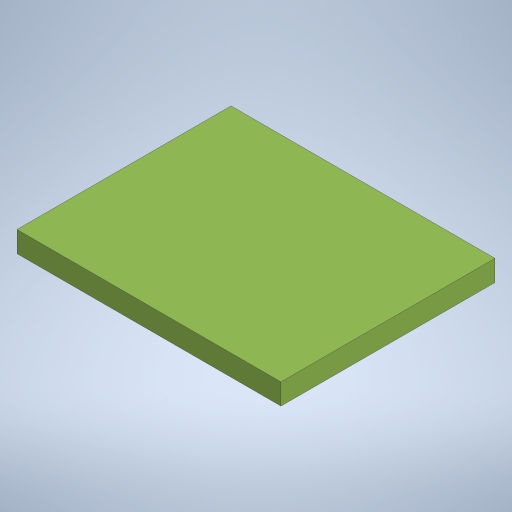
# Autodesk Inventor part: sensor
Saved by Autodesk Inventor 2023 (Build 270158000, 158)
## iProperties
Created: 2023-10-14
Part Number: sensor
Material: Generic
Document SubType Name: Modeling
Designer: Gage
Density: 1 g/cm^3
Appearance: Default
Author: Gage
Autodesk Inventor part; units mm, degrees
ref_plane "YZ Plane" through (0, 0, 0) normal (1, 0, 0) x (0, 1, 0)
ref_plane "XZ Plane" through (0, 0, 0) normal (0, 1, 0) x (-1, 0, 0)
ref_plane "XY Plane" through (0, 0, 0) normal (0, 0, 1) x (1, 0, 0)
sketch "Sketch1" plane through (0, 0, 0) normal (0, 1, 0) x (-1, 0, 0)
  line L0 (9.6647, -7.8359) -> (-9.6647, -7.8359)
  line L1 (-9.6647, -7.8359) -> (-9.6647, 7.8359)
  line L2 (-9.6647, 7.8359) -> (9.6647, 7.8359)
  line L3 (9.6647, 7.8359) -> (9.6647, -7.8359)
  point P0 (0, 0)
  point P1 (0, -7.8359)
  point P2 (-9.6647, 0)
  dimension "d2" = 19.3294
  dimension "d3" = 15.6718
  constraints: 8 end point, 2 midpoint, 2 parallel, 1 horizontal, 1 horizontal alignment, 1 perpendicular, 1 vertical alignment
  measures "d2" distance of L1.end L2.end
  measures "d3" distance of L0.end L1.end
extrude "Extrusion1" add sketch "Sketch1" along normal blind 1.5367
body "Solid1"
